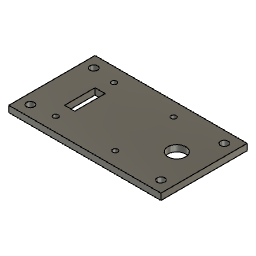
display-mount v1 (Autodesk Fusion 360 design; units mm, degrees)
Autodesk Fusion 360 part; units mm, degrees
sketch "Skizze1" plane through (0, 0, 0) normal (0, 0, 1) x (1, 0, 0)
  line L0 (0, 0) -> (60, 0)
  line L1 (60, 0) -> (60, 34)
  line L2 (60, 34) -> (0, 34)
  line L3 (0, 34) -> (0, 0)
  circle A0 centre (4, 4.5) radius 1.5
  circle A1 centre (55.5, 4.5) radius 1.5
  circle A2 centre (55.5, 4.5) radius 1.5
  circle A3 centre (4, 4.5) radius 1.5
  line L4 (0, 0) -> (60, 0)
  circle A4 centre (55.5, 29.5) radius 1.5
  circle A5 centre (4, 29.5) radius 1.5
  circle A6 centre (55.5, 29.5) radius 1.5
  circle A7 centre (4, 29.5) radius 1.5
  circle A8 centre (13, 28.5) radius 1
  circle A9 centre (13, 5.5) radius 1
  circle A10 centre (36.5, 5.5) radius 1
  circle A11 centre (36.5, 28.5) radius 1
  line L5 (11, 23) -> (15, 23)
  line L6 (15, 23) -> (15, 11)
  line L7 (15, 11) -> (11, 11)
  line L8 (11, 11) -> (11, 23)
  circle A12 centre (49, 17.25) radius 3.5
  point P0 (51.5, 0)
  point P1 (51.5, 0)
  point P2 (51.5, 0)
  point P3 (51.5, 0)
  dimension "d1" = 60
  dimension "d2" = 34
  dimension "d3" = 3
  dimension "d4" = 3
  dimension "d5" = 60
  dimension "d6" = 3
  dimension "d7" = 3
  dimension "d8" = 3
  dimension "d9" = 3
  dimension "d10" = 3
  dimension "d11" = 3
  dimension "d12" = 2
  dimension "d13" = 2
  dimension "d14" = 2
  dimension "d15" = 2
  dimension "d16" = 7
  constraint horizontal L0
  constraint vertical L1
  constraint horizontal L2
  constraint vertical L3
  constraint coincident L0.start L3.end
  constraint coincident P3 P2
  constraint horizontal L4
  constraint horizontal L5
  constraint vertical L6
  constraint horizontal L7
  constraint vertical L8
  measures "d1" distance of L0.start L0.end
  measures "d2" distance of L0.start L2.end
  measures "d3" diameter of A0
  measures "d4" diameter of A1
  measures "d5" distance of L0.end L0.start
  measures "d6" diameter of A3
  measures "d7" diameter of A2
  measures "d8" diameter of A5
  measures "d9" diameter of A4
  measures "d10" diameter of A7
  measures "d11" diameter of A6
  measures "d12" diameter of A8
  measures "d13" diameter of A9
  measures "d14" diameter of A11
  measures "d15" diameter of A10
  measures "d16" diameter of A12
extrude "Extrusion1" add sketch "Skizze1" along normal blind 2.5
